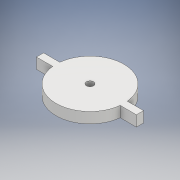
# Autodesk Inventor part: RescueKitThrow_bottom
Saved by Autodesk Inventor 2018.3 (Build 223284000, 284)
## iProperties
Created: 2019-02-10
Part Number: RescueKitThrow_bottom
Material: ABS プラスチック
Document SubType Name: Modeling
Designer: shun2
Density: 1.06 g/cm^3
Appearance: 滑らか - 白
Author: shun2
Autodesk Inventor part; units mm, degrees
ref_plane "YZ Plane" through (0, 0, 0) normal (1, 0, 0) x (0, 1, 0)
ref_plane "XZ Plane" through (0, 0, 0) normal (0, 1, 0) x (-1, 0, 0)
ref_plane "XY Plane" through (0, 0, 0) normal (0, 0, 1) x (1, 0, 0)
sketch "スケッチ1" plane through (0, 0, 0) normal (0, 0, 1) x (1, 0, 0)
  line L0 (-14, 1) -> (-9.4472, 1)
  line L1 (-9.4472, -1) -> (-14, -1)
  line L2 (-14, -1) -> (-14, 1)
  line L3 (14, 1) -> (9.4472, 1)
  line L4 (9.4472, -1) -> (14, -1)
  arc A0 (9.4472, 1) -> (-9.4472, 1) centre (0, 0) ccw
  arc A1 (-9.4472, -1) -> (9.4472, -1) centre (0, 0) ccw
  line L5 (14, -1) -> (14, 1)
  circle A2 centre (0, 0) radius 1
  dimension "d3" = 2
  constraints: 12 end point, 4 point on circle, 3 centre point, 2 coincident, 2 horizontal, 2 parallel, 1 vertical
  measures "d3" diameter of A2
extrude "押し出し1" add sketch "スケッチ1" along normal blind 3
